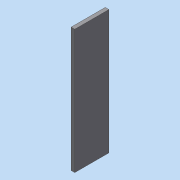
# Autodesk Inventor part: Bearing-Side
Saved by Autodesk Inventor 2016 SP1 (Build 200210100, 210)
## iProperties
Created: 2016-03-02
Part Number: Bearing-Side
Material: Generic
Document SubType Name: Modeling
Designer: Mohamed A.
Density: 1 g/cm^3
Appearance: Default
Author: Mohamed A.
Autodesk Inventor part; units mm, degrees
ref_plane "YZ Plane" through (0, 0, 0) normal (1, 0, 0) x (0, 1, 0)
ref_plane "XZ Plane" through (0, 0, 0) normal (0, 1, 0) x (-1, 0, 0)
ref_plane "XY Plane" through (0, 0, 0) normal (0, 0, 1) x (1, 0, 0)
sketch "Sketch2" plane through (0, 0, 0) normal (1, 0, 0) x (0, 1, 0)
  line L0 (14, -51) -> (11, -51)
  line L1 (-14, 51) -> (-11, 51)
  line L2 (14, 51) -> (14, 48)
  line L3 (-14, 51) -> (-14, 48)
  line L4 (14, -48) -> (11, -48)
  line L5 (11, -51) -> (11, -48)
  line L6 (0, -71.4) -> (0, 71.4) construction
  line L7 (3.975, -51) -> (3.975, -48)
  line L8 (-3.975, -51) -> (-3.975, -48)
  line L9 (1.5, -48) -> (1.5, -46)
  line L10 (1.5, -46) -> (2.65, -46)
  line L11 (2.65, -46) -> (2.65, -43.6)
  line L12 (2.65, -43.6) -> (1.5, -43.6)
  line L13 (1.5, -43.6) -> (1.5, -43)
  line L14 (1.5, -43) -> (-1.5, -43)
  line L15 (-1.5, -43) -> (-1.5, -43.6)
  line L16 (-1.5, -43.6) -> (-2.65, -43.6)
  line L17 (-2.65, -43.6) -> (-2.65, -46)
  line L18 (-2.65, -46) -> (-1.5, -46)
  line L19 (-1.5, -46) -> (-1.5, -48)
  line L20 (11, -51) -> (-14, -51)
  line L21 (1.5, -48) -> (-14, -48)
  line L22 (3.975, -48) -> (1.5, -48)
  line L23 (11, -48) -> (3.975, -48)
  line L24 (-19.6, 0) -> (19.6, 0) construction
  line L25 (-11, -51) -> (-11, -48)
  line L26 (14, 48) -> (11, 48)
  line L27 (11, 51) -> (11, 48)
  line L28 (3.975, 51) -> (3.975, 48)
  line L29 (-3.975, 51) -> (-3.975, 48)
  line L30 (1.5, 48) -> (1.5, 46)
  line L31 (1.5, 46) -> (2.65, 46)
  line L32 (2.65, 46) -> (2.65, 43.6)
  line L33 (2.65, 43.6) -> (1.5, 43.6)
  line L34 (1.5, 43.6) -> (1.5, 43)
  line L35 (1.5, 43) -> (-1.5, 43)
  line L36 (-1.5, 43) -> (-1.5, 43.6)
  line L37 (-1.5, 43.6) -> (-2.65, 43.6)
  line L38 (-2.65, 43.6) -> (-2.65, 46)
  line L39 (-2.65, 46) -> (-1.5, 46)
  line L40 (-1.5, 46) -> (-1.5, 48)
  line L41 (1.5, 48) -> (-14, 48)
  line L42 (3.975, 48) -> (1.5, 48)
  line L43 (11, 48) -> (3.975, 48)
  line L44 (-11, 51) -> (-11, 48)
  line L45 (3.975, 51) -> (11, 51)
  line L46 (-3.975, 51) -> (3.975, 51)
  line L47 (11, -48) -> (11, -1.5)
  line L48 (-11, 48) -> (-11, 18)
  line L49 (14, 21) -> (11, 21) construction
  line L50 (14, -21) -> (11, -21) construction
  line L51 (14, 18) -> (11, 18)
  line L52 (14, -18) -> (11, -18)
  line L53 (14, -3.975) -> (11, -3.975)
  line L54 (14, 3.975) -> (11, 3.975)
  line L55 (11, 1.5) -> (9, 1.5)
  line L56 (9, 1.5) -> (9, 2.65)
  line L57 (9, 2.65) -> (6.6, 2.65)
  line L58 (6.6, 2.65) -> (6.6, 1.5)
  line L59 (6.6, 1.5) -> (6, 1.5)
  line L60 (6, 1.5) -> (6, -1.5)
  line L61 (6, -1.5) -> (6.6, -1.5)
  line L62 (6.6, -1.5) -> (6.6, -2.65)
  line L63 (6.6, -2.65) -> (9, -2.65)
  line L64 (9, -2.65) -> (9, -1.5)
  line L65 (11, -1.5) -> (9, -1.5)
  line L66 (14, -3.975) -> (14, -18)
  line L67 (14, 3.975) -> (14, -3.975)
  line L68 (11, 1.5) -> (11, 48)
  line L69 (11, -1.5) -> (11, 1.5)
  line L70 (-14, 18) -> (-11, 18)
  line L71 (-14, -18) -> (-11, -18)
  line L72 (-14, -3.975) -> (-11, -3.975)
  line L73 (-14, 3.975) -> (-11, 3.975)
  line L74 (-11, 1.5) -> (-9, 1.5)
  line L75 (-9, 1.5) -> (-9, 2.65)
  line L76 (-9, 2.65) -> (-6.6, 2.65)
  line L77 (-6.6, 2.65) -> (-6.6, 1.5)
  line L78 (-6.6, 1.5) -> (-6, 1.5)
  line L79 (-6, 1.5) -> (-6, -1.5)
  line L80 (-6, -1.5) -> (-6.6, -1.5)
  line L81 (-6.6, -1.5) -> (-6.6, -2.65)
  line L82 (-6.6, -2.65) -> (-9, -2.65)
  line L83 (-9, -2.65) -> (-9, -1.5)
  line L84 (-11, -1.5) -> (-9, -1.5)
  line L85 (-14, 3.975) -> (-14, -3.975)
  line L86 (-14, -3.975) -> (-14, -18)
  line L87 (-14, 18) -> (-14, 3.975)
  line L88 (-14, -18) -> (-14, -51)
  line L89 (14, -18) -> (14, -51)
  line L90 (14, 18) -> (14, 3.975)
  line L91 (-11, -3.975) -> (-11, -18)
  line L92 (-11, -18) -> (-11, -48)
  line L93 (-11, 18) -> (-11, 3.975)
  line L94 (14, 48) -> (14, 18)
  line L95 (-14, 48) -> (-14, 18)
  line L96 (-11, 51) -> (-3.975, 51)
  line L97 (11, 51) -> (14, 51)
  line L98 (-11, 3.975) -> (-11, 1.5)
  line L99 (-11, 1.5) -> (-11, -1.5)
  line L100 (-11, -1.5) -> (-11, -3.975)
  point P0 (0, 0)
  dimension "d5" = 3
  dimension "d6" = 3
  dimension "d8" = 2.4
  dimension "d9" = 5.3
  dimension "d10" = 3
  dimension "d11" = 2
  dimension "d12" = 5
  dimension "d13" = 7.95
  dimension "d14" = 28
  dimension "d15" = 102
  dimension "d17" = 42
  dimension "d18" = 3
  dimension "d19" = 3
  dimension "d20" = 2
  dimension "d21" = 5
  dimension "d22" = 2.4
  dimension "d23" = 5.3
  dimension "d24" = 3
  dimension "d25" = 7.95
  constraints: 198 end point, 65 point on line, 47 perpendicular, 42 symmetric about line, 32 parallel, 4 vertical, 3 horizontal, 10 other
  measures "d5" distance between parallel lines of L0 L4
  measures "d6" distance between parallel lines of L5 L2
  measures "d8" distance between parallel lines of L10 L12
  measures "d9" distance between parallel lines of L17 L11
  measures "d10" distance between parallel lines of L15 L13
  measures "d11" distance between parallel lines of L4 L10
  measures "d12" distance between parallel lines of L4 L14
  measures "d13" distance between parallel lines of L8 L7
  measures "d14" distance between parallel lines of L3 L2
  measures "d15" distance between parallel lines of L20 L1
  measures "d17" distance between parallel lines of L49 L50
  measures "d18" distance between parallel lines of L49 L51
  measures "d19" distance between parallel lines of L50 L52
  measures "d20" distance between parallel lines of L47 L56
  measures "d21" distance between parallel lines of L47 L60
  measures "d22" distance between parallel lines of L58 L56
  measures "d23" distance between parallel lines of L63 L57
  measures "d24" distance between parallel lines of L65 L55
  measures "d25" distance between parallel lines of L53 L54
extrude "Extrusion1" add sketch "Sketch2" along normal blind 3 contours L20 L7 L23 L5 | L23 L22 L9 L10 L11 L12 L13 L14 L15 L16 L17 L18 L19 L21 L92 L91 L100 L84 L83 L82 L81 L80 L79 L78 L77 L76 L75 L74 L98 L93 L48 L41 L40 L39 L38 L37 L36 L35 L34 L33 L32 L31 L30 L42 L43 L68 L55 L56 L57 L58 L59 L60 L61 L62 L63 L64 L65 L47 | L52 L47 L53 L66 | L20 L25 L21 L8 | L54 L68 L51 L90 | L71 L86 L72 L91 | L43 L28 L45 L27 | L87 L70 L93 L73 | L29 L41 L44 L96
equation "\"d13\" = 1.5 * d9"
equation "\"d25\" = 1.5 * d23"
body "Solid1"
